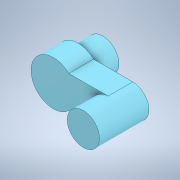
# Autodesk Inventor part: Component31
Saved by Autodesk Inventor 2022 (Build 260153000, 153)
## iProperties
Created: 2022-01-29
Part Number: Component31
Material: Generic
Document SubType Name: Modeling
Designer: Administrator
Density: 1 g/cm^3
Appearance: Default
Title: Component31
Author: Administrator
Autodesk Inventor part; units mm, degrees
ref_plane "YZ Plane" through (0, 0, 0) normal (1, 0, 0) x (0, 1, 0)
ref_plane "XZ Plane" through (0, 0, 0) normal (0, 1, 0) x (-1, 0, 0)
ref_plane "XY Plane" through (0, 0, 0) normal (0, 0, 1) x (1, 0, 0)
sketch "Sketch2" plane through (0, 0, 0) normal (0, 0, 1) x (1, 0, 0)
  circle A0 centre (-3.175, -1.5465) radius 3.25
  line L0 (-0.0625, 1.7035) -> (7.8834, 1.7035)
  arc A1 (-0.0625, 1.7035) -> (-0.0625, -4.7965) centre (-3.175, -1.5465) ccw
  circle A2 centre (7.8834, -1.5465) radius 3.25
  line L1 (-11.3863, -1.5465) -> (20.6188, -1.5465) construction
  line L2 (-0.0625, -4.7965) -> (7.8834, -4.7965)
  point P0 (9.6395, 1.7844)
  dimension "d6" = 11.0584
  dimension "d7" = 6.5
  dimension "d8" = 6.5
  dimension "d9" = 9
  constraints: 6 end point, 3 horizontal, 2 centre point, 2 coincident, 2 point on circle, 2 point on line, 2 symmetric about line, 3 other
  measures "d6" distance of point (7.883, -1.547) point (-3.175, -1.547)
  measures "d7" distance between parallel lines of L0 L2
  measures "d8" diameter of A0
  measures "d9" diameter of A1
extrude "Extrusion1" add sketch "Sketch2" along normal blind 5 contours A0 | L0 A2 L2 A1 | A2
extrude "Extrusion2" add sketch "Sketch2" against normal blind 5 contours A0
sketch "Sketch3" plane through (0, 0, 5) normal (0, 0, 1) x (1, 0, 0)
  circle A0 centre (7.8834, -1.5465) radius 3.25 projected
  point P0 (0, 0)
extrude "Extrusion3" add sketch "Sketch3" along normal blind 5
equation "\"d7\" = width"
equation "\"d8\" = width"
equation "\"d9\" = R1"
equation "\"d0\" = thickness"
equation "\"d2\" = thickness"
equation "\"d4\" = thickness"
equation "\"R\" = 6.5"
equation "\"thickness\" = 5"
equation "\"width\" = 6.5"
equation "\"R1\" = 9"
body "Solid1"
